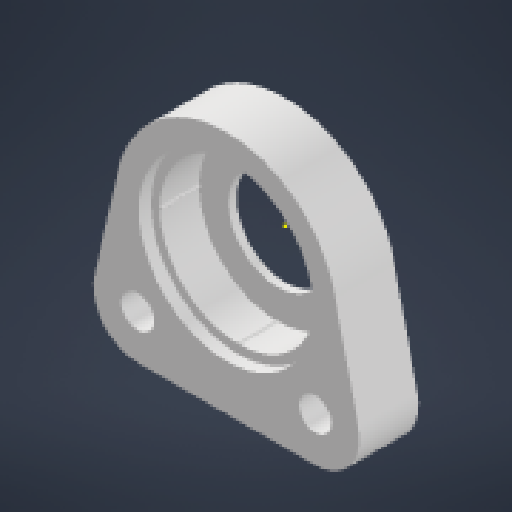
# Autodesk Inventor part: Conveyor Bearing Housing
Saved by Autodesk Inventor 2025 (Build 290162000, 162)
## iProperties
Created: 2024-12-26
Part Number: Conveyor Bearing Housing
Material: Generic
Document SubType Name: Modeling
Designer: Juan
Density: 1 g/cm^3
Appearance: Default
Author: Juan
Autodesk Inventor part; units mm, degrees
ref_plane "YZ Plane" through (0, 0, 0) normal (1, 0, 0) x (0, 1, 0)
ref_plane "XZ Plane" through (0, 0, 0) normal (0, 1, 0) x (-1, 0, 0)
ref_plane "XY Plane" through (0, 0, 0) normal (0, 0, 1) x (1, 0, 0)
sketch "Sketch1" plane through (0, 0, 0) normal (0, 0, 1) x (1, 0, 0)
  arc A0 (-5.827627, -9.579088) -> (-0.250527, -11.231057) centre (0.025157, -0.060123) ccw
  arc A1 (0.25, -11.209713) -> (5.829601, -9.582326) centre (0.025157, -0.060123) ccw
  line L0 (0.46552, -11.403002) -> (0, -10.9855)
  line L1 (0, -10.9855) -> (-0.46552, -11.403002)
  arc A2 (-11.176173, -0.249433) -> (-9.579088, -5.827627) centre (0.025157, -0.060123) ccw
  line L2 (-11.403002, -0.46552) -> (-10.9855, 0)
  line L3 (-10.9855, 0) -> (-11.403002, 0.46552)
  arc A3 (-9.579088, 5.827627) -> (-11.209713, 0.25) centre (0, 0) ccw
  arc A4 (5.827627, 9.579088) -> (0.25, 11.209713) centre (0, 0) ccw
  line L4 (0, 10.9855) -> (0.46552, 11.403002)
  line L5 (-0.46552, 11.403002) -> (0, 10.9855)
  arc A5 (-0.25, 11.209713) -> (-5.827627, 9.579088) centre (0, 0) ccw
  arc A6 (11.209713, 0.25) -> (9.579088, 5.827627) centre (0, 0) ccw
  line L6 (11.403002, 0.46552) -> (10.9855, 0)
  line L7 (10.9855, 0) -> (11.403002, -0.46552)
  arc A7 (9.579088, -5.827627) -> (11.209713, -0.25) centre (0, 0) ccw
  arc A8 (7.230816, -10.196338) -> (10.196338, -7.230816) centre (0, 0) ccw
  arc A9 (-10.196338, -7.230816) -> (-7.230816, -10.196338) centre (0, 0) ccw
  arc A10 (-7.230816, 10.196338) -> (-10.196338, 7.230816) centre (0, 0) ccw
  circle A11 centre (0, 0) radius 12.5
  circle A12 centre (12.7, -12.7) radius 2.3241
  circle A13 centre (-12.7, -12.7) radius 2.3241
  line L8 (-19.05, -12.7) -> (19.05, -12.7) construction
  line L9 (-12.7, -19.05) -> (12.7, -19.05)
  line L10 (12.7, -6.35) -> (-12.7, -6.35)
  arc A14 (-12.7, -6.35) -> (-12.7, -19.05) centre (-12.7, -12.7) ccw
  arc A15 (12.7, -19.05) -> (12.7, -6.35) centre (12.7, -12.7) ccw
  circle A16 centre (0, 0) radius 11.2125
  circle A17 centre (0, 0) radius 15.875
  line L11 (15.560093, 3.146287) -> (18.887388, -11.272158)
  line L12 (0, -10.9855) -> (0, -12.5)
  line L13 (-15.560093, 3.146287) -> (-18.887388, -11.272158)
  point P0 (-0.46552, -11.403002)
  point P1 (-11.403002, -0.46552)
  point P2 (0, -12.7)
  point P3 (10.196338, -7.230816)
  point P4 (7.230816, -10.196338)
  point P5 (-7.230816, -10.196338)
  point P6 (-10.196338, -7.230816)
  point P7 (-10.196338, 7.230816)
  point P8 (-7.230816, 10.196338)
  point P9 (-0.25, -11.209713)
  point P10 (0.25, -11.209713)
  point P11 (9.579088, -5.827627)
  point P12 (9.579088, 5.827627)
  point P13 (-5.827627, 9.579088)
  point P14 (-9.579088, 5.827627)
  point P15 (-11.209713, -0.25)
  dimension "d0" = 25
  dimension "d9" = 31.75
  dimension "d1" = 4.6482
  dimension "d2" = 4.6482
  dimension "d4" = 6.35
  dimension "d5" = 6.35
  dimension "d6" = 12.7
  dimension "d8" = 25.4
  constraints: 29 point on circle, 26 end point, 15 centre point, 5 tangent, 3 coincident, 2 point on line, 2 symmetric about line, 1 midpoint, 1 parallel, 1 vertical, 16 other
  measures "d1" diameter of A12
  measures "d2" diameter of A13
  measures "d4" distance of A13.centre L8.start
  measures "d5" distance of A12.centre L8.end
  measures "d6" diameter of A15
  measures "d8" distance of A12.centre A13.centre
extrude "Extrusion1" add sketch "Sketch1" along normal blind 12.7 contours L10 A14 A17 A15 A11 A10 | A11 A9 A8 L10 A15 A17 A12 A13 A14 | A17 A13 A12 A15 L9 A14 | A14 L13 A17 | A17 L11 A15
extrude "Extrusion2" add sketch "Sketch1" along normal blind 10.9982 contours A16 L1 A0 | A0 L1 A16 L12 A11 A9 L10 | A16 L10 L0 L1 | A16 L2 L3 A3 A5 L5 L4 A4 A6 L6 L7 A7 L10 | L10 A11 A10 A16 A7 A6 A4 A5 A3 | L1 L12 A16 | L10 A11 A8 L12 A16 | L0 A16 L12 | A16 L3 L2 | L7 L6 A16 | A16 L4 L5
sketch "Sketch1 outline for Extrusion3" plane through (0, 0, 0) normal (0, 0, 1) x (1, 0, 0)
  arc A0 (-11.209713, -0.25) -> (-0.25, -11.209713) centre (0, 0) ccw
  line L0 (-10.9855, 0) -> (-11.209713, -0.25)
  line L1 (-11.209713, 0.25) -> (-10.9855, 0)
  arc A1 (-9.579088, 5.827627) -> (-11.209713, 0.25) centre (0, 0) ccw
  arc A2 (-5.827627, 9.579088) -> (-9.579088, 5.827627) centre (0, 0) ccw
  arc A3 (-0.25, 11.209713) -> (-5.827627, 9.579088) centre (0, 0) ccw
  line L2 (0, 10.9855) -> (-0.25, 11.209713)
  line L3 (0.25, 11.209713) -> (0, 10.9855)
  arc A4 (5.827627, 9.579088) -> (0.25, 11.209713) centre (0, 0) ccw
  arc A5 (9.579088, 5.827627) -> (5.827627, 9.579088) centre (0, 0) ccw
  arc A6 (11.209713, 0.25) -> (9.579088, 5.827627) centre (0, 0) ccw
  line L4 (10.9855, 0) -> (11.209713, 0.25)
  line L5 (11.209713, -0.25) -> (10.9855, 0)
  arc A7 (9.579088, -5.827627) -> (11.209713, -0.25) centre (0, 0) ccw
  arc A8 (0.25, -11.209713) -> (9.579088, -5.827627) centre (0, 0) ccw
  line L6 (0, -10.9855) -> (0.25, -11.209713)
  line L7 (-0.25, -11.209713) -> (0, -10.9855)
extrude "Extrusion3" cut sketch "Sketch1 outline for Extrusion3" along normal blind 10.9982
sketch "Sketch2" plane through (0, 0, 0) normal (0, 0, -1) x (-1, 0, 0)
  arc A0 (-0.25, 11.209713) -> (-11.209713, 0.25) centre (0, 0) ccw
  arc A1 (11.209713, 0.25) -> (0.25, 11.209713) centre (0, 0) ccw
  line L0 (0, 10.9855) -> (0.25, 11.209713)
  line L1 (-0.25, 11.209713) -> (0, 10.9855)
  line L2 (11.209713, 0.25) -> (10.9855, 0)
  line L3 (10.9855, 0) -> (11.209713, -0.25)
  arc A2 (0.25, -11.209713) -> (11.209713, -0.25) centre (0, 0) ccw
  line L4 (0.25, -11.209713) -> (0, -10.9855)
  line L5 (0, -10.9855) -> (-0.25, -11.209713)
  arc A3 (-11.209713, -0.25) -> (-0.25, -11.209713) centre (0, 0) ccw
  line L6 (-11.209713, -0.25) -> (-10.9855, 0)
  line L7 (-10.9855, 0) -> (-11.209713, 0.25)
  circle A4 centre (0, 0) radius 6.9977
  point P0 (0, 0)
  dimension "d16" = 13.9954
  constraints: 1 centre point, 1 coincident
  measures "d16" diameter of A4
extrude "Extrusion4" add sketch "Sketch2" against normal blind 5.3848
sketch "Sketch3" plane through (0, 0, 0) normal (0, 0, -1) x (-1, 0, 0)
  circle A0 centre (0, 0) radius 6.9977
  arc A1 (12.7, -19.05) -> (18.887388, -11.272158) centre (12.7, -12.7) ccw
  line L0 (15.560093, 3.146287) -> (18.887388, -11.272158)
  arc A2 (15.560093, 3.146287) -> (-15.560093, 3.146287) centre (0, 0) ccw
  line L1 (-18.887388, -11.272158) -> (-15.560093, 3.146287)
  arc A3 (-18.887388, -11.272158) -> (-12.7, -19.05) centre (-12.7, -12.7) ccw
  line L2 (12.7, -19.05) -> (-12.7, -19.05)
  circle A4 centre (12.7, -12.7) radius 2.3241
  circle A5 centre (-12.7, -12.7) radius 2.3241
  point P0 (0, 0)
extrude "Extrusion5" cut sketch "Sketch3" against normal blind 4.233333
sketch "Sketch4" plane through (0, 0, 4.233333) normal (0, 0, -1) x (-1, 0, 0)
  point P0 (0, 0)
sketch "Sketch5" plane through (0, 0, 4.233333) normal (0, 0, -1) x (-1, 0, 0)
  point P0 (0, 0)
body "Solid1"
